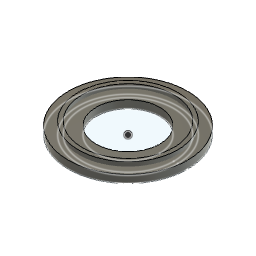
USBCDiscs v1 (Autodesk Fusion 360 design; units mm, degrees)
Autodesk Fusion 360 part; units mm, degrees
sketch "Sketch1" plane through (0, 0, 0) normal (0, 1, 0) x (1, 0, 0)
  circle A0 centre (0, 0) radius 15
  circle A1 centre (0, 0) radius 8
  circle A2 centre (0, 0) radius 12.5
  circle A3 centre (0, 0) radius 11.5
  dimension "d1" = 30
  dimension "d2" = 16
  dimension "d5" = 25
  dimension "d6" = 23
  constraint coincident A0.centre A1.centre
  constraint concentric A1 A3
  measures "d1" diameter of A0
  measures "d2" diameter of A1
  measures "d5" diameter of A2
  measures "d6" diameter of A3
extrude "Extrude2" add sketch "Sketch1" along normal blind 3 contours A2 makes body 1
extrude "Extrude1" add sketch "Sketch1" along normal blind 2 separate body contours A0 | A2 | A3 makes body 2
